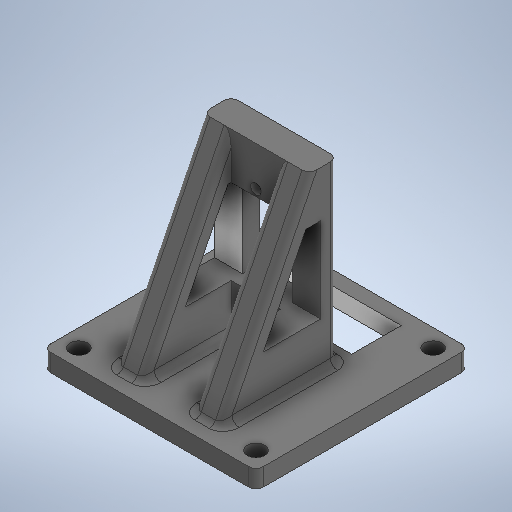
# Autodesk Inventor part: Servo_podstawa
Saved by Autodesk Inventor 2025.2 (Build 292293000, 293)
## iProperties
Created: 2025-11-25
Part Number: Servo_podstawa
Material: Ogólny
Document SubType Name: Modeling
Designer: juras
Density: 1 g/cm^3
Appearance: Domyślna
Author: juras
Autodesk Inventor part; units mm, degrees
ref_plane "YZ Plane" through (0, 0, 0) normal (1, 0, 0) x (0, 1, 0)
ref_plane "XZ Plane" through (0, 0, 0) normal (0, 1, 0) x (-1, 0, 0)
ref_plane "XY Plane" through (0, 0, 0) normal (0, 0, 1) x (1, 0, 0)
sketch "Szkic1" plane through (0, 0, 0) normal (0, 1, 0) x (-1, 0, 0)
  line L0 (30, 30) -> (-30, 30)
  line L1 (-30, 30) -> (-30, -30)
  line L2 (-30, -30) -> (30, -30)
  line L3 (30, -30) -> (30, 30)
  line L4 (30, 30) -> (-30, -30) construction
  line L5 (-30, 30) -> (30, -30) construction
  point P0 (0, 0)
  dimension "d0" = 60
  dimension "d1" = 60
  constraints: 12 end point, 2 midpoint, 2 parallel, 1 horizontal, 1 perpendicular
  measures "d0" distance of L2.end L1.end
  measures "d1" distance of L1.end L0.end
extrude "Wyciągnięcie proste1" add sketch "Szkic1" along normal mid plane 5
sketch "Szkic2" plane through (0, 2.5, 0) normal (0, 1, 0) x (1, 0, 0)
  line L0 (-25, -25) -> (25, -25)
  line L1 (25, -25) -> (25, 25)
  line L2 (25, 25) -> (-25, 25)
  line L3 (-25, 25) -> (-25, -25)
  line L4 (-25, -25) -> (25, 25) construction
  line L5 (25, -25) -> (-25, 25) construction
  point P0 (0, 0)
  dimension "d4" = 50
  dimension "d5" = 50
  constraints: 12 end point, 4 coincident, 2 midpoint, 2 parallel, 1 horizontal, 1 perpendicular
  measures "d4" distance of L2.end L1.end
  measures "d5" distance of L1.end L0.end
hole "Otwór1" at (-25, 2.5, -25) at (25, 2.5, -25) at (-25, 2.5, 25) at (25, 2.5, 25) direction (0, -1, 0) diameter 5 depth 25 tip angle 118
fillet "Zaokrąglenie1" radius 2 4 edges at (-30, 0, -30) (-30, 0, 30) (30, 0, 30) (30, 0, -30)
sketch "Szkic5" plane through (0, 2.5, 0) normal (0, 1, 0) x (1, 0, 0)
  line L0 (0, 0) -> (7, 0)
  line L1 (0, 0) -> (-7, 0)
  line L2 (-7, 0) -> (-15, 0)
  line L3 (-15, 0) -> (-15, -25)
  line L4 (-15, -25) -> (-7, -25)
  line L5 (-7, -25) -> (-7, 0)
  line L6 (7, 0) -> (15, 0)
  line L7 (15, 0) -> (15, -25)
  line L8 (15, -25) -> (7, -25)
  line L9 (7, -25) -> (7, 0)
  line L10 (-15, 0) -> (15, 0)
  line L11 (15, 0) -> (15, 8)
  line L12 (15, 8) -> (-15, 8)
  line L13 (-15, 8) -> (-15, 0)
  dimension "d14" = 7
  dimension "d15" = 7
  dimension "d16" = 8
  dimension "d17" = 25
  dimension "d18" = 8
  dimension "d19" = 25
  dimension "d20" = 30
  dimension "d21" = 8
  constraints: 28 end point, 6 parallel, 5 horizontal, 3 perpendicular
  measures "d14" distance of L0.start L0.end
  measures "d15" distance of L0.start L1.end
  measures "d16" distance of L4.end L3.end
  measures "d17" distance of L3.end L2.end
  measures "d18" distance of L7.end L8.end
  measures "d19" distance of L6.end L7.end
  measures "d20" distance of L12.end L11.end
  measures "d21" distance of L11.end L10.end
extrude "Wyciągnięcie proste2" add sketch "Szkic5" along normal blind 50
sketch "Szkic8" plane through (-7, 2.5, 0) normal (0, 0, 1) x (1, 0, 0)
  point P0 (7, -2.5)
sketch "Szkic9" plane through (-7, 2.5, 0) normal (0, 0, 1) x (1, 0, 0)
  line L0 (0, 37) -> (14, 37)
  line L1 (14, 37) -> (14, 13)
  line L2 (14, 13) -> (0, 13)
  line L3 (0, 13) -> (0, 37)
  line L4 (0, 50) -> (14, 50) projected
  line L5 (14, 0) -> (0, 0) projected
  line L6 (0, 0) -> (0, 50) projected
  line L7 (14, 0) -> (14, 50) projected
  point P0 (7, -2.5)
  point P1 (7, 37)
  point P2 (0, 37)
  point P3 (14, 37)
  dimension "d24" = 13
  dimension "d25" = 13
  dimension "d26" = 0
  dimension "d27" = 0
  constraints: 8 end point, 2 parallel, 1 horizontal, 1 midpoint, 1 perpendicular
  measures "d24" distance from line of L4 point (7, 37)
  measures "d25" distance between parallel lines of L5 L2
  measures "d26" distance between parallel lines of L6 L3
  measures "d27" distance between parallel lines of L1 L7
extrude "Wyciągnięcie proste3" cut sketch "Szkic9" against normal blind 10 contours L0 L1 L2 L3
sketch "Szkic10" plane through (-7, 2.5, 0) normal (0, 0, 1) x (1, 0, 0)
  point P0 (7, -2.5)
sketch "Szkic11" plane through (-7, 52.5, 0) normal (0, 0, 1) x (1, 0, 0)
  line L0 (14, -37) -> (0, -37) projected
  line L1 (7, -37) -> (7, -38.9)
  point P0 (7, -52.5)
  dimension "d30" = 1.9
  constraints: 2 end point, 1 midpoint, 1 vertical
  measures "d30" distance of L1.start L1.end
hole "Otwór2" at (0, 13.6, 0) direction (0, 0, -1) diameter 3 depth 25 tip angle 118
sketch "Szkic12" plane through (-7, 52.5, 0) normal (0, 0, 1) x (1, 0, 0)
  line L0 (0, -13) -> (14, -13) projected
  line L1 (7, -13) -> (7, -11.1)
  point P0 (7, -52.5)
  dimension "d38" = 1.9
  constraints: 2 end point, 1 midpoint, 1 vertical
  measures "d38" distance of L1.start L1.end
hole "Otwór3" at (0, 41.4, 0) direction (0, 0, -1) diameter 3 depth 25 tip angle 118
sketch "Szkic13" plane through (-7, 2.5, 25) normal (1, 0, 0) x (0, 0, -1)
  line L0 (0, 50) -> (25, 50) projected
  line L1 (25, 50) -> (0, 0)
  line L2 (0, 0) -> (0, 50) projected
  line L3 (0, 0) -> (0, 50)
  line L4 (0, 50) -> (25, 50)
  point P0 (25, -2.5)
  constraints: 6 end point, 1 collinear, 1 perpendicular, 1 point on line
extrude "Wyciągnięcie proste4" cut sketch "Szkic13" against normal blind 10
sketch "Szkic14" plane through (7, 2.5, 0) normal (-1, 0, 0) x (0, 0, 1)
  line L0 (0, 50) -> (25, 50) projected
  line L1 (0, 50) -> (25, 50)
  line L2 (25, 0) -> (0, 0) projected
  line L3 (25, 50) -> (25, 0)
  line L4 (0, 37) -> (0, 50) projected
  line L5 (25, 0) -> (0, 50)
  point P0 (0, -2.5)
  constraints: 6 end point, 1 collinear, 1 perpendicular
extrude "Wyciągnięcie proste5" cut sketch "Szkic14" against normal blind 10
fillet "Zaokrąglenie2" radius 2 6 edges at (-15, 27.5, -8) (-15, 27.5, 12.5) (-7, 27.5, 12.5) (7, 27.5, 12.5) (15, 27.5, 12.5) (15, 27.5, -8)
sketch "Szkic15" plane through (-15, 2.5, -6) normal (-1, 0, 0) x (0, 0, 1)
  point P0 (6, -2.5)
sketch "Szkic16" plane through (-15, 2.5, -6) normal (-1, 0, 0) x (0, 0, 1)
  line L0 (6, 13) -> (-2, 13) projected
  line L1 (7.4872, 13) -> (18.9736, 13)
  line L2 (18.9736, 13) -> (6.9494, 37)
  line L3 (6.9494, 37) -> (2.7554, 37)
  line L4 (2.7554, 37) -> (2.7554, 13)
  line L5 (2.7554, 13) -> (7.4872, 13)
  line L6 (0, 0) -> (0, 50) projected
  line L7 (0, 50) -> (3.7639, 50) projected
  line L8 (3.7639, 50) -> (28.7639, 0) projected
  point P0 (6, -2.5)
  point P1 (4.8524, 37)
  point P2 (12.9615, 25)
  point P3 (2.7554, 13)
  dimension "d51" = 2.7554
  dimension "d52" = 13
  dimension "d53" = 2.9538
  dimension "d54" = 26.611
  constraints: 10 end point, 2 midpoint, 2 perpendicular, 2 point on line, 1 horizontal, 1 parallel
  measures "d51" distance between parallel lines of L4 L6
  measures "d52" distance from line of L7 point (4.852, 37)
  measures "d53" distance from line of L8 point (12.961, 25)
  measures "d54" angle of L6 L2
extrude "Wyciągnięcie proste6" cut sketch "Szkic16" along normal through all both and the other way through all
fillet "Zaokrąglenie3" radius 2 14 edges at (-14.4142, 2.5, -7.4142) (0, 2.5, -8) (14.4142, 2.5, -7.4142) (15, 2.5, 8.382) (14.4142, 2.5, 24.3451) (11, 2.5, 25) (7.5858, 2.5, 24.3451) (7, 2.5, 11.382) (-14.4142, 2.5, 24.3451) (-11, 2.5, 25) (-7.5858, 2.5, 24.3451) (-7, 2.5, 11.382) (-15, 2.5, 8.382) (0, 2.5, 0)
sketch "Szkic17" plane through (0, 2.5, 0) normal (0, 1, 0) x (1, 0, 0)
  line L0 (15, 26) -> (-15, 26)
  line L1 (-15, 26) -> (-15, 12)
  line L2 (-15, 12) -> (15, 12)
  line L3 (15, 12) -> (15, 26)
  line L4 (15, 26) -> (-15, 12) construction
  line L5 (-15, 26) -> (15, 12) construction
  line L6 (30, -28) -> (30, 28) projected
  line L7 (-30, 28) -> (-30, -28) projected
  line L8 (-13, 8) -> (13, 8) projected
  line L9 (28, 30) -> (-28, 30) projected
  point P0 (0, 0)
  point P1 (0, 19)
  dimension "d58" = 15
  dimension "d59" = 15
  dimension "d60" = 4
  dimension "d61" = 4
  constraints: 12 end point, 2 midpoint, 2 parallel, 1 horizontal, 1 perpendicular
  measures "d58" distance between parallel lines of L3 L6
  measures "d59" distance between parallel lines of L7 L1
  measures "d60" distance between parallel lines of L8 L2
  measures "d61" distance between parallel lines of L9 L0
extrude "Wyciągnięcie proste7" cut sketch "Szkic17" against normal blind 10
